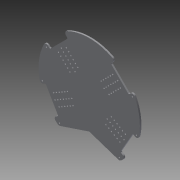
# Autodesk Inventor part: Bottom Plate
Saved by Autodesk Inventor 2015 (Build 190159000, 159)
## iProperties
Created: 2016-08-02
Part Number: Bottom Plate
Material: Generic
Document SubType Name: Modeling
Designer: James Yelland
Density: 1 g/cm^3
Appearance: Default
Author: James Yelland
Autodesk Inventor part; units mm, degrees
ref_plane "YZ Plane" through (0, 0, 0) normal (1, 0, 0) x (0, 1, 0)
ref_plane "XZ Plane" through (0, 0, 0) normal (0, 1, 0) x (-1, 0, 0)
ref_plane "XY Plane" through (0, 0, 0) normal (0, 0, 1) x (1, 0, 0)
sketch "Sketch1" plane through (0, 0, 0) normal (0, 1, 0) x (-1, 0, 0)
  line L0 (73.6122, -42.5) -> (62.1122, -62.4186)
  line L1 (62.8442, -65.1506) -> (65.5625, -66.72)
  line L2 (73.6122, -42.5) -> (85.1122, -22.5814)
  line L3 (87.8442, -21.8494) -> (90.5625, -23.4188)
  line L4 (-73.6122, -42.5) -> (-62.1122, -62.4186)
  line L5 (-62.8442, -65.1506) -> (-65.5625, -66.72)
  line L6 (-73.6122, -42.5) -> (-85.1122, -22.5814)
  line L7 (-87.8442, -21.8494) -> (-90.5625, -23.4188)
  line L8 (-60.1041, 60.1041) -> (-76.3675, 43.8406)
  line L9 (-79.196, 43.8406) -> (-81.4154, 46.0601)
  line L10 (-60.1041, 60.1041) -> (-43.8406, 76.3675)
  line L11 (-43.8406, 79.196) -> (-46.0601, 81.4154)
  line L12 (60.1041, 60.1041) -> (43.8406, 76.3675)
  line L13 (43.8406, 79.196) -> (46.0601, 81.4154)
  line L14 (60.1041, 60.1041) -> (76.3675, 43.8406)
  line L15 (79.196, 43.8406) -> (81.4154, 46.0601)
  circle A0 centre (68.0696, -39.3) radius 1.65
  circle A1 centre (62.5703, -36.125) radius 1.65
  circle A2 centre (57.0711, -32.95) radius 1.65
  circle A3 centre (51.5718, -29.775) radius 1.65
  circle A4 centre (46.0726, -26.6) radius 1.65
  circle A5 centre (40.5733, -23.425) radius 1.65
  circle A6 centre (35.074, -20.25) radius 1.65
  circle A7 centre (32.4636, -31.2714) radius 1.7
  circle A8 centre (37.9629, -34.4464) radius 1.7
  circle A9 centre (43.4621, -37.6214) radius 1.7
  circle A10 centre (48.9614, -40.7964) radius 1.7
  circle A11 centre (54.4607, -43.9714) radius 1.7
  circle A12 centre (59.9599, -47.1464) radius 1.7
  circle A13 centre (70.8099, -28.3536) radius 1.7
  circle A14 centre (65.3107, -25.1786) radius 1.7
  circle A15 centre (59.8114, -22.0036) radius 1.7
  circle A16 centre (54.3121, -18.8286) radius 1.7
  circle A17 centre (48.8129, -15.6536) radius 1.7
  circle A18 centre (43.3136, -12.4786) radius 1.7
  circle A19 centre (-68.0696, -39.3) radius 1.65
  circle A20 centre (-62.5703, -36.125) radius 1.65
  circle A21 centre (-57.0711, -32.95) radius 1.65
  circle A22 centre (-51.5718, -29.775) radius 1.65
  circle A23 centre (-46.0726, -26.6) radius 1.65
  circle A24 centre (-40.5733, -23.425) radius 1.65
  circle A25 centre (-35.074, -20.25) radius 1.65
  circle A26 centre (-43.3136, -12.4786) radius 1.7
  circle A27 centre (-48.8129, -15.6536) radius 1.7
  circle A28 centre (-54.3121, -18.8286) radius 1.7
  circle A29 centre (-59.8114, -22.0036) radius 1.7
  circle A30 centre (-65.3107, -25.1786) radius 1.7
  circle A31 centre (-70.8099, -28.3536) radius 1.7
  circle A32 centre (-59.9599, -47.1464) radius 1.7
  circle A33 centre (-54.4607, -43.9714) radius 1.7
  circle A34 centre (-48.9614, -40.7964) radius 1.7
  circle A35 centre (-43.4621, -37.6214) radius 1.7
  circle A36 centre (-37.9629, -34.4464) radius 1.7
  circle A37 centre (-32.4636, -31.2714) radius 1.7
  circle A38 centre (-55.5786, 55.5786) radius 1.65
  circle A39 centre (-51.0885, 51.0885) radius 1.65
  circle A40 centre (-46.5983, 46.5983) radius 1.65
  circle A41 centre (-42.1082, 42.1082) radius 1.65
  circle A42 centre (-37.6181, 37.6181) radius 1.65
  circle A43 centre (-33.128, 33.128) radius 1.65
  circle A44 centre (-28.6378, 28.6378) radius 1.65
  circle A45 centre (-23.2638, 38.608) radius 1.7
  circle A46 centre (-27.7539, 43.0982) radius 1.7
  circle A47 centre (-32.2441, 47.5883) radius 1.7
  circle A48 centre (-36.7342, 52.0784) radius 1.7
  circle A49 centre (-41.2243, 56.5685) radius 1.7
  circle A50 centre (-45.7145, 61.0587) radius 1.7
  circle A51 centre (-61.0587, 45.7145) radius 1.7
  circle A52 centre (-56.5685, 41.2243) radius 1.7
  circle A53 centre (-52.0784, 36.7342) radius 1.7
  circle A54 centre (-47.5883, 32.2441) radius 1.7
  circle A55 centre (-43.0982, 27.7539) radius 1.7
  circle A56 centre (-38.608, 23.2638) radius 1.7
  circle A57 centre (55.5786, 55.5786) radius 1.65
  circle A58 centre (51.0885, 51.0885) radius 1.65
  circle A59 centre (46.5983, 46.5983) radius 1.65
  circle A60 centre (42.1082, 42.1082) radius 1.65
  circle A61 centre (37.6181, 37.6181) radius 1.65
  circle A62 centre (33.128, 33.128) radius 1.65
  circle A63 centre (28.6378, 28.6378) radius 1.65
  circle A64 centre (38.608, 23.2638) radius 1.7
  circle A65 centre (43.0982, 27.7539) radius 1.7
  circle A66 centre (47.5883, 32.2441) radius 1.7
  circle A67 centre (52.0784, 36.7342) radius 1.7
  circle A68 centre (56.5685, 41.2243) radius 1.7
  circle A69 centre (61.0587, 45.7145) radius 1.7
  circle A70 centre (45.7145, 61.0587) radius 1.7
  circle A71 centre (41.2243, 56.5685) radius 1.7
  circle A72 centre (36.7342, 52.0784) radius 1.7
  circle A73 centre (32.2441, 47.5883) radius 1.7
  circle A74 centre (27.7539, 43.0982) radius 1.7
  circle A75 centre (23.2638, 38.608) radius 1.7
  arc A76 (97.9605, -20.0933) -> (89.422, 44.7627) centre (0, 0) ccw
  arc A77 (44.7627, 89.422) -> (-44.7627, 89.422) centre (0, 0) ccw
  arc A78 (-89.422, 44.7627) -> (-97.9605, -20.0933) centre (0, 0) ccw
  arc A79 (90.5625, -23.4188) -> (97.9605, -20.0933) centre (93.0625, -19.0886) ccw
  arc A80 (66.3816, -74.7896) -> (65.5625, -66.72) centre (63.0625, -71.0502) ccw
  arc A81 (-65.5625, -66.72) -> (-66.3816, -74.7896) centre (-63.0625, -71.0502) ccw
  arc A82 (-97.9605, -20.0933) -> (-90.5625, -23.4188) centre (-93.0625, -19.0886) ccw
  arc A83 (-81.4154, 46.0601) -> (-89.422, 44.7627) centre (-84.9509, 42.5245) ccw
  arc A84 (-44.7627, 89.422) -> (-46.0601, 81.4154) centre (-42.5245, 84.9509) ccw
  arc A85 (46.0601, 81.4154) -> (44.7627, 89.422) centre (42.5245, 84.9509) ccw
  arc A86 (89.422, 44.7627) -> (81.4154, 46.0601) centre (84.9509, 42.5245) ccw
  arc A87 (62.1122, -62.4186) -> (62.8442, -65.1506) centre (63.8442, -63.4186) ccw
  arc A88 (87.8442, -21.8494) -> (85.1122, -22.5814) centre (86.8442, -23.5814) ccw
  arc A89 (76.3675, 43.8406) -> (79.196, 43.8406) centre (77.7817, 45.2548) ccw
  arc A90 (43.8406, 79.196) -> (43.8406, 76.3675) centre (45.2548, 77.7817) ccw
  arc A91 (-43.8406, 76.3675) -> (-43.8406, 79.196) centre (-45.2548, 77.7817) ccw
  arc A92 (-79.196, 43.8406) -> (-76.3675, 43.8406) centre (-77.7817, 45.2548) ccw
  arc A93 (-85.1122, -22.5814) -> (-87.8442, -21.8494) centre (-86.8442, -23.5814) ccw
  arc A94 (-62.8442, -65.1506) -> (-62.1122, -62.4186) centre (-63.8442, -63.4186) ccw
  circle A95 centre (-84.9509, 42.5245) radius 1.6
  circle A96 centre (-93.0625, -19.0886) radius 1.6
  circle A97 centre (84.9509, 42.5245) radius 1.6
  circle A98 centre (93.0625, -19.0886) radius 1.6
  line L16 (0, -60) -> (-57.4738, -79.1579)
  line L17 (0, -60) -> (57.4738, -79.1579)
  arc A99 (62.1631, -78.3311) -> (66.3816, -74.7896) centre (0, 0) ccw
  arc A100 (-66.3816, -74.7896) -> (-62.1631, -78.3311) centre (0, 0) ccw
  arc A101 (57.4738, -79.1579) -> (62.1631, -78.3311) centre (59.0549, -74.4145) ccw
  arc A102 (-62.1631, -78.3311) -> (-57.4738, -79.1579) centre (-59.0549, -74.4145) ccw
  circle A103 centre (59.0549, -74.4145) radius 1.6
  circle A104 centre (-59.0549, -74.4145) radius 1.6
  point P0 (61.1122, -64.1506)
  point P1 (71.3525, -70.0629)
  point P2 (86.1122, -20.8494)
  point P3 (96.3525, -26.7617)
  point P4 (-61.1122, -64.1506)
  point P5 (-71.3525, -70.0629)
  point P6 (-86.1122, -20.8494)
  point P7 (-96.3525, -26.7617)
  point P8 (-77.7817, 42.4264)
  point P9 (-86.143, 50.7877)
  point P10 (-50.7877, 86.143)
  point P11 (42.4264, 77.7817)
  point P12 (50.7877, 86.143)
  point P13 (77.7817, 42.4264)
  point P14 (86.143, 50.7877)
  point P15 (60, -80)
  point P16 (-60, -80)
  dimension "d5" = 25
  dimension "d6" = 25
  dimension "d8" = 25
  dimension "d11" = 25
  dimension "d14" = 25
  dimension "d15" = 25
  dimension "d22" = 5
  dimension "d26" = 3.2
  dimension "d27" = 3.2
  dimension "d28" = 3.2
  dimension "d29" = 3.2
  dimension "d35" = 5
  dimension "d36" = 3.2
  dimension "d37" = 3.2
  constraints: 105 centre point, 54 point on circle, 36 end point, 34 tangent, 27 point on line, 15 equal radius, 10 coincident, 7 perpendicular
  measures "d5" distance of L0.start point (61.112, -64.151)
  measures "d6" distance of L0.start point (86.112, -20.849)
  measures "d8" distance of L4.start point (-61.112, -64.151)
  measures "d11" distance of L8.start point (-77.782, 42.426)
  measures "d14" distance of L12.start point (42.426, 77.782)
  measures "d15" distance of L12.start point (77.782, 42.426)
  measures "d22" radius of A79
  measures "d26" diameter of A95
  measures "d27" diameter of A96
  measures "d28" diameter of A97
  measures "d29" diameter of A98
  measures "d35" radius of A101
  measures "d36" diameter of A103
  measures "d37" diameter of A104
extrude "Extrusion1" add sketch "Sketch1" along normal blind 3
body "Solid1"
